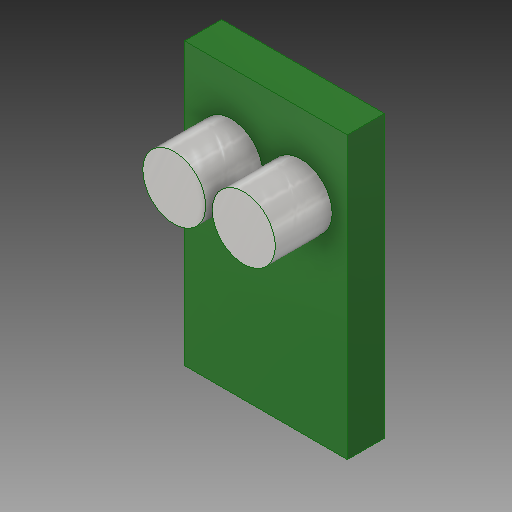
# Autodesk Inventor part: サイドワインダーマイクロ2
Saved by Autodesk Inventor 2020 (Build 240168000, 168)
## iProperties
Created: 2018-11-28
Part Number: サイドワインダーマイクロ2
Material: 一般
Document SubType Name: Modeling
Designer: 雪村
Mass: 26 g
Surface Area: 26.8323 cm^2
Volume: 5.05387 cm^3
Density: 5.14457 g/cm^3
Appearance: 深緑
Author: 雪村
Autodesk Inventor part; units mm, degrees
ref_plane "YZ Plane" through (0, 0, 0) normal (1, 0, 0) x (0, 1, 0)
ref_plane "XZ Plane" through (0, 0, 0) normal (0, 1, 0) x (-1, 0, 0)
ref_plane "XY Plane" through (0, 0, 0) normal (0, 0, 1) x (1, 0, 0)
sketch "スケッチ1" plane through (0, 0, 0) normal (0, 0, 1) x (1, 0, 0)
  line L0 (0, 0) -> (62, 0) construction
  line L1 (62, 0) -> (62, -62) construction
  line L2 (62, -62) -> (0, -62) construction
  line L3 (0, -62) -> (0, 0) construction
  line L4 (20.6, -15.3248) -> (42.6, -15.3248)
  line L5 (42.6, -15.3248) -> (42.6, -53.3248)
  line L6 (42.6, -53.3248) -> (20.6, -53.3248)
  line L7 (20.6, -53.3248) -> (20.6, -15.3248)
  circle A0 centre (26.9, -25.5248) radius 4.25
  circle A1 centre (36.3, -25.5248) radius 4.25
  dimension "d1" = 22
  dimension "d2" = 38
  dimension "d3" = 62
  dimension "d12" = 15.3248
  dimension "d16" = 20.6
  dimension "d17" = 8.5
  dimension "d18" = 8.5
  dimension "d19" = 6.3
  dimension "d25" = 10.2
  dimension "d31" = 6.3
  constraints: 8 end point, 3 horizontal, 2 centre point, 2 vertical, 1 horizontal alignment, 2 other
  measures "d1" distance of L5.end L6.end
  measures "d2" distance of L4.end L5.end
  measures "d3" distance of L0.end L1.end
  measures "d12" distance between parallel lines of L0 L4
  measures "d16" distance between parallel lines of L7 L3
  measures "d17" diameter of A0
  measures "d18" diameter of A1
  measures "d19" distance from line of L7 A0.centre
  measures "d25" distance from line of L4 A0.centre
  measures "d31" distance from line of L5 A1.centre
extrude "押し出し1" add sketch "スケッチ1" along normal blind 5
sketch "スケッチ2" plane through (0, 0, 0) normal (0, 0, -1) x (-1, 0, 0)
  circle A0 centre (-36.3, -25.5248) radius 4.25 projected
  circle A1 centre (-26.9, -25.5248) radius 4.25 projected
  point P0 (0, 0)
extrude "押し出し2" add sketch "スケッチ2" against normal blind 12.7
equation "\"d17\" = d18"
equation "\"d31\" = d19"
